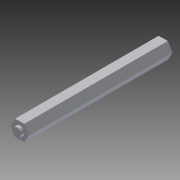
# Autodesk Inventor part: 4.5 hex shaft
Saved by Autodesk Inventor 2014 SP1 (Build 180222100, 222)
## iProperties
Created: 2013-11-21
Part Number: 4.5 hex shaft
Material: Aluminum 6061
Document SubType Name: Modeling
Designer: Arpan
Density: 2.71 g/cm^3
Appearance: Aluminum - Flat
Mass: 38.4958 g
Surface Area: 47.5572 cm^2
Volume: 14.2051 cm^3
d0: 0.500 in
d1: 4.000 in
d2: 0.00 deg
d3: 0.010 in
d4: 0.00 deg
Author: Arpan
Autodesk Inventor part; units mm, degrees
ref_plane "YZ Plane" through (0, 0, 0) normal (1, 0, 0) x (0, 1, 0)
ref_plane "XZ Plane" through (0, 0, 0) normal (0, 1, 0) x (-1, 0, 0)
ref_plane "XY Plane" through (0, 0, 0) normal (0, 0, 1) x (1, 0, 0)
sketch "Sketch1" plane through (0, 0, 0) normal (0, 0, 1) x (1, 0, 0)
  line L0 (-3.7629, 6.2932) -> (3.5686, 6.4054)
  line L1 (3.5686, 6.4054) -> (7.3315, 0.1122)
  line L2 (7.3315, 0.1122) -> (3.7629, -6.2932)
  line L3 (3.7629, -6.2932) -> (-3.5686, -6.4054)
  line L4 (-3.5686, -6.4054) -> (-7.3315, -0.1122)
  line L5 (-7.3315, -0.1122) -> (-3.7629, 6.2932)
  point P0 (0, 0)
  point P1 (0, 0)
  dimension "d0" = 12.7
  constraints: 12 end point, 1 coincident, 13 other
  measures "d0" distance between parallel lines of L0 L3
extrude "Extrusion1" add sketch "Sketch1" along normal blind 101.6
sketch "Sketch2" plane through (0, 0, 101.6) normal (0, 0, 1) x (1, 0, 0)
  circle A0 centre (0, 0) radius 4.1084
  constraints: 1 centre point, 1 coincident
extrude "Extrusion2" add sketch "Sketch2" along normal blind 0.254
sketch "Sketch3" plane through (0, 0, 101.6) normal (0, 0, 1) x (1, 0, 0)
  line L0 (3.5686, 6.4054) -> (-3.7629, 6.2932) projected
  line L1 (-3.7629, 6.2932) -> (-7.3315, -0.1122) projected
  line L2 (-7.3315, -0.1122) -> (-3.5686, -6.4054) projected
  line L3 (-3.5686, -6.4054) -> (3.7629, -6.2932) projected
  line L4 (3.7629, -6.2932) -> (7.3315, 0.1122) projected
  line L5 (7.3315, 0.1122) -> (3.5686, 6.4054) projected
extrude "Extrusion3" add sketch "Sketch3" along normal blind 12.7
sketch "Sketch4" plane through (0, 0, 114.3) normal (0, 0, 1) x (1, 0, 0)
  circle A0 centre (0, 0) radius 3.5518
  constraints: 1 centre point, 1 coincident
extrude "Extrusion4" add sketch "Sketch4" along normal blind 2.54
body "Solid1"
